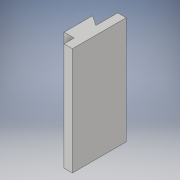
# Autodesk Inventor part: Inner Rail 1
Saved by Autodesk Inventor 2019 (Build 230136000, 136)
## iProperties
Created: 2019-03-02
Part Number: Inner Rail 1
Material: Generic
Document SubType Name: Modeling
Designer: Jared
Density: 1 g/cm^3
Appearance: Default
Author: Jared
Autodesk Inventor part; units mm, degrees
ref_plane "YZ Plane" through (0, 0, 0) normal (1, 0, 0) x (0, 1, 0)
ref_plane "XZ Plane" through (0, 0, 0) normal (0, 1, 0) x (-1, 0, 0)
ref_plane "XY Plane" through (0, 0, 0) normal (0, 0, 1) x (1, 0, 0)
sketch "Sketch2" plane through (0, 0, 0) normal (0, 1, 0) x (-1, 0, 0)
  line L0 (0, 0) -> (2.5, 0)
  line L1 (0, 0) -> (0, -16)
  line L2 (0, -16) -> (2.5, -16)
  line L3 (2.5, 0) -> (2.5, -3)
  line L4 (2.5, -16) -> (2.5, -9.5)
  line L5 (2.5, -3) -> (5.5, -3)
  line L6 (5.5, -3) -> (5.5, -11.5)
  line L7 (2.5, -9.5) -> (5.5, -11.5)
  dimension "d1" = 2.5
  dimension "d2" = 16
  dimension "d3" = 3
  dimension "d4" = 6.5
  dimension "d5" = 3
  dimension "d6" = 8.5
  constraints: 16 end point, 3 vertical, 2 horizontal, 2 perpendicular, 1 parallel
  measures "d1" distance of L0.start L0.end
  measures "d2" distance of L0.start L1.end
  measures "d3" distance of L0.end L3.end
  measures "d4" distance of L2.end L4.end
  measures "d5" distance of L3.end L5.end
  measures "d6" distance of L5.end L6.end
extrude "Extrusion1" add sketch "Sketch2" along normal blind 32
body "Solid1"
